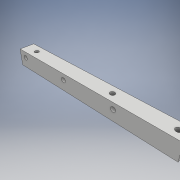
# Autodesk Inventor part: support
Saved by Autodesk Inventor 2017 (Build 210142000, 142)
## iProperties
Created: 2017-08-21
Part Number: support
Material: Generic
Document SubType Name: Modeling
Designer: ndz
Density: 1 g/cm^3
Appearance: Default
Author: ndz
Autodesk Inventor part; units mm, degrees
ref_plane "YZ Plane" through (0, 0, 0) normal (1, 0, 0) x (0, 1, 0)
ref_plane "XZ Plane" through (0, 0, 0) normal (0, 1, 0) x (-1, 0, 0)
ref_plane "XY Plane" through (0, 0, 0) normal (0, 0, 1) x (1, 0, 0)
sketch "Sketch1" plane through (0, 0, 0) normal (0, 0, 1) x (1, 0, 0)
  line L0 (0, 0) -> (110, 0)
  line L1 (110, 0) -> (110, 10)
  line L2 (110, 10) -> (0, 10)
  line L3 (0, 10) -> (0, 0)
  circle A0 centre (10, 5) radius 1.6
  circle A1 centre (70, 5) radius 1.6
  circle A2 centre (105, 5) radius 1.6
  dimension "d0" = 110
  dimension "d1" = 10
  dimension "d2" = 90
  dimension "d3" = 110
  dimension "d4" = 3.2
  dimension "d6" = 3.2
  dimension "d7" = 3.2
  dimension "d8" = 60
  dimension "d9" = 35
  constraints: 8 end point, 3 centre point, 2 perpendicular, 1 horizontal
  measures "d0" distance of L0.start L0.end
  measures "d1" distance of L0.end L1.end
  measures "d2" angle of L1 L0
  measures "d3" distance of L1.end L2.end
  measures "d4" diameter of A0
  measures "d6" diameter of A1
  measures "d7" diameter of A2
  measures "d8" distance of A1.centre A0.centre
  measures "d9" distance of A2.centre A1.centre
extrude "Extrusion1" add sketch "Sketch1" along normal blind 11
sketch "Sketch2" plane through (0, 0, 0) normal (0, -1, 0) x (1, 0, 0)
  line L0 (0, 0) -> (0, 11) projected
  line L1 (110, 0) -> (110, 11) projected
  line L2 (0, 0) -> (110, 0) projected
  circle A0 centre (5, 7) radius 1.6
  circle A1 centre (75, 7) radius 1.6
  circle A2 centre (40, 7) radius 1.6
  dimension "d13" = 3.2
  dimension "d14" = 5
  dimension "d15" = 3.2
  dimension "d16" = 70
  dimension "d17" = 3.2
  dimension "d18" = 35
  constraints: 3 centre point
  measures "d13" diameter of A0
  measures "d14" distance from line of L0 A0.centre
  measures "d15" diameter of A1
  measures "d16" distance of A0.centre A1.centre
  measures "d17" diameter of A2
  measures "d18" distance of A0.centre A2.centre
extrude "Extrusion2" cut sketch "Sketch2" against normal blind 10
body "Solid1"
